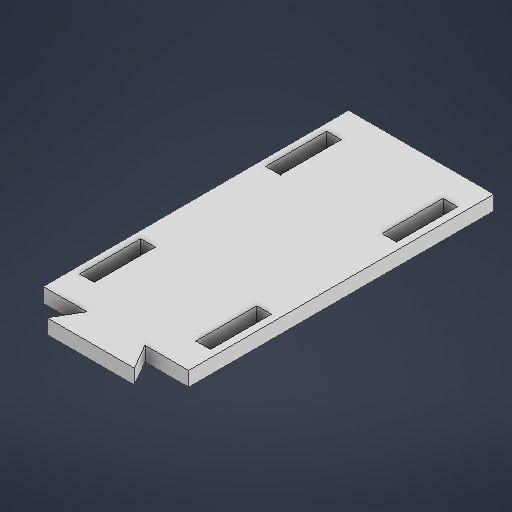
# Autodesk Inventor part: inslide1
Saved by Autodesk Inventor 2026.2 (Build 302298000, 298)
## iProperties
Created: 2026-04-17
Part Number: inslide1
Material: Generic
Document SubType Name: Modeling
Designer: danda
Density: 1 g/cm^3
Appearance: Default
Author: danda
Autodesk Inventor part; units mm, degrees
ref_plane "YZ Plane" through (0, 0, 0) normal (1, 0, 0) x (0, 1, 0)
ref_plane "XZ Plane" through (0, 0, 0) normal (0, 1, 0) x (-1, 0, 0)
ref_plane "XY Plane" through (0, 0, 0) normal (0, 0, 1) x (1, 0, 0)
sketch "Sketch1" plane through (0, 0, 0) normal (0, 0, 1) x (1, 0, 0)
  line L0 (9.4704, 26.4594) -> (59.4704, 26.4594)
  line L1 (59.4704, 26.4594) -> (59.4704, 21.4594)
  line L2 (59.4704, 21.4594) -> (9.4704, 21.4594)
  line L3 (9.4704, 21.4594) -> (9.4704, 26.4594)
  point P0 (0, 0)
  dimension "d0" = 50
  dimension "d1" = 5
  constraints: 8 end point, 2 parallel, 1 horizontal, 1 perpendicular
  measures "d0" distance of L1.end L2.end
  measures "d1" distance of L0.end L1.end
extrude "Extrusion1" add sketch "Sketch1" along normal blind 105
sketch "Sketch2" plane through (9.4704, 26.4594, 0) normal (0, 1, 0) x (1, 0, 0)
  line L0 (0, -105) -> (50, -105) projected
  line L1 (0, 0) -> (50, 0) projected
  line L2 (0, -105) -> (50, -105)
  line L3 (50, -105) -> (50, 0)
  line L4 (50, 0) -> (0, 0)
  line L5 (0, 0) -> (0, -105)
  line L6 (2.5, -95) -> (7.5, -95)
  line L7 (7.5, -95) -> (7.5, -74)
  line L8 (7.5, -74) -> (2.5, -74)
  line L9 (2.5, -74) -> (2.5, -95)
  line L10 (42.5, -95) -> (47.5, -95)
  line L11 (47.5, -95) -> (47.5, -74)
  line L12 (47.5, -74) -> (42.5, -74)
  line L13 (42.5, -74) -> (42.5, -95)
  line L14 (42.5, -31) -> (47.5, -31)
  line L15 (47.5, -31) -> (47.5, -10)
  line L16 (47.5, -10) -> (42.5, -10)
  line L17 (42.5, -10) -> (42.5, -31)
  line L18 (2.5, -31) -> (7.5, -31)
  line L19 (7.5, -31) -> (7.5, -10)
  line L20 (7.5, -10) -> (2.5, -10)
  line L21 (2.5, -10) -> (2.5, -31)
  line L22 (15, -105) -> (10, -113.6603)
  line L23 (15, -105) -> (25, -105) construction
  line L24 (10, -113.6603) -> (40, -113.6603)
  line L25 (40, -113.6603) -> (35, -105)
  point P0 (-9.4704, 0)
  dimension "d4" = 5
  dimension "d5" = 21
  dimension "d6" = 5
  dimension "d7" = 21
  dimension "d8" = 5
  dimension "d9" = 21
  dimension "d10" = 5
  dimension "d11" = 21
  dimension "d12" = 2.5
  dimension "d13" = 2.5
  dimension "d14" = 2.5
  dimension "d15" = 2.5
  dimension "d16" = 10
  dimension "d17" = 10
  dimension "d18" = 10
  dimension "d19" = 10
  dimension "d22" = 10
  dimension "d23" = 120
  dimension "d24" = 30
  dimension "d25" = 10
  dimension "d26" = 15
  constraints: 48 end point, 10 parallel, 7 horizontal, 5 perpendicular, 2 point on line, 1 equal length
  measures "d4" distance of L8.end L7.end
  measures "d5" distance of L7.end L6.end
  measures "d6" distance of L12.end L11.end
  measures "d7" distance of L11.end L10.end
  measures "d8" distance of L16.end L15.end
  measures "d9" distance of L15.end L14.end
  measures "d10" distance of L20.end L19.end
  measures "d11" distance of L19.end L18.end
  measures "d12" distance between parallel lines of L5 L9
  measures "d13" distance between parallel lines of L5 L21
  measures "d14" distance between parallel lines of L3 L11
  measures "d15" distance between parallel lines of L3 L15
  measures "d16" distance between parallel lines of L0 L6
  measures "d17" distance between parallel lines of L1 L20
  measures "d18" distance between parallel lines of L1 L16
  measures "d19" distance between parallel lines of L0 L10
  measures "d22" distance of L22.start L22.end
  measures "d23" angle of L22 L23
  measures "d24" distance of L22.end L24.end
  measures "d25" distance of L24.end L25.end
  measures "d26" distance of L0.start L22.start
extrude "Extrusion2" cut sketch "Sketch2" against normal blind 105 contours L9 L8 L7 L6 | L13 L12 L11 L10 | L17 L16 L15 L14 | L21 L20 L19 L18
extrude "Extrusion3" add sketch "Sketch2" against normal blind 5 contours L0 L25 L24 L22
equation "\"d13\" = d12"
equation "\"d14\" = d12"
equation "\"d15\" = d12"
equation "\"d17\" = d16"
equation "\"d18\" = d16"
equation "\"d19\" = d16"
body "Solid1"
